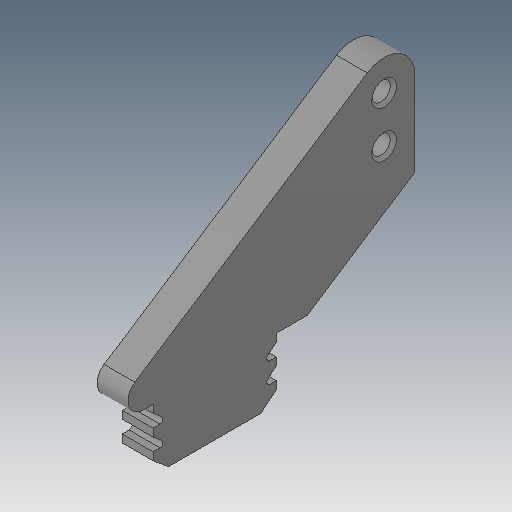
# Autodesk Inventor part: control_horn
Saved by Autodesk Inventor 2019 (Build 230136000, 136)
## iProperties
Created: 2022-04-02
Part Number: control_horn
Material: ABS Plastic
Document SubType Name: Modeling
Designer: solyo
Density: 1.06 g/cm^3
Appearance: Smooth - Medium Gray
Mass: 0.317862 g
Surface Area: 4.33026 cm^2
Volume: 0.29987 cm^3
Author: solyo
Autodesk Inventor part; units mm, degrees
ref_plane "YZ Plane" through (0, 0, 0) normal (1, 0, 0) x (0, 1, 0)
ref_plane "XZ Plane" through (0, 0, 0) normal (0, 1, 0) x (-1, 0, 0)
ref_plane "XY Plane" through (0, 0, 0) normal (0, 0, 1) x (1, 0, 0)
sketch "Sketch1" plane through (0, 0, 0) normal (1, 0, 0) x (0, 1, 0)
  line L0 (0, 0) -> (11.6754, -17.9077)
  line L1 (10, -21) -> (4.5638, -21)
  line L2 (0, -14) -> (4.5638, -21)
  line L3 (0, 0) -> (0, -4)
  line L4 (0, -4) -> (-4, -4)
  line L5 (-4, -4) -> (-4, -12)
  line L6 (-4, -12) -> (0, -12)
  line L7 (0, -12) -> (0, -14)
  arc A0 (10, -21) -> (11.6754, -17.9077) centre (10, -19) ccw
  point P0 (13.6915, -21)
  point P1 (7, -19)
  dimension "d26" = 8
  dimension "d31" = 4
  dimension "d32" = 2
  dimension "d43" = 2
  dimension "d44" = 5
  dimension "d45" = 10
  dimension "d64" = 3
  dimension "d65" = 4
  constraints: 16 end point, 3 parallel, 3 point on line, 2 horizontal, 2 point on circle, 2 tangent, 1 centre point, 1 coincident, 1 collinear, 1 vertical
  measures "d26" distance of L4.end L5.end
  measures "d31" distance between parallel lines of L3 L5
  measures "d32" distance of L6.end L2.start
  measures "d43" radius of A0
  measures "d44" vertical distance of L2.start A0.centre
  measures "d45" horizontal distance of L0.start point (10, -19)
  measures "d64" distance of A0.centre point (7, -19)
  measures "d65" distance of L0.start L3.end
extrude "Extrusion1" add sketch "Sketch1" along normal blind 2
hole "Hole3" at (0, 10, -19) at (0, 7, -19) direction (1, 0, 0) diameter 1.2 end through all
fillet "Fillet3" radius 1 1 edges at (1, 0, 0)
chamfer "Chamfer2" distance 0.2 angle 45 4 edges at (2, 10, -19.6) (0, 10, -19.6) (0, 7, -19.6) (2, 7, -19.6)
ref_plane "Work Plane1" through (0, -4, -8) normal (0, 0, -1) x (-1, 0, 0)
sketch "Sketch4" plane through (2, 0, 0) normal (1, 0, 0) x (0, 0, -1)
  arc A0 (2.8186, 1.8377) -> (3.3648, 0) centre (3.3648, 1) ccw projected
  line L0 (3.3648, 0) -> (4, 0) projected
  line L1 (4, 0) -> (4, -4) projected
  line L2 (4, -4) -> (12, -4) projected
  line L3 (12, -4) -> (12, 0) projected
  line L4 (12, 0) -> (14, 0) projected
  line L5 (14, 0) -> (21, 4.5638) projected
  line L6 (21, 4.5638) -> (21, 10) projected
  arc A1 (21, 10) -> (17.9077, 11.6754) centre (19, 10) ccw projected
  line L7 (17.9077, 11.6754) -> (2.8186, 1.8377) projected
  circle A2 centre (19, 10) radius 0.8 projected
  line L8 (4, 0) -> (12, 0)
  line L9 (12, -4) -> (4, -4) projected
  line L10 (5, -4) -> (4, -3.1667)
  line L11 (4, -4) -> (4, 0) projected
  line L12 (4, -2.6667) -> (5, -2.6667)
  line L13 (5, -2.6667) -> (4, -1.8333)
  line L14 (4, -1.3333) -> (5, -1.3333)
  line L15 (5, -1.3333) -> (4, -0.5)
  line L16 (4, -0.5) -> (4, 0)
  line L17 (4, -0.5) -> (4, -1.3333)
  line L18 (4, -1.8333) -> (4, -2.6667)
  line L19 (4, -3.1667) -> (4, -4)
  line L20 (4, -4) -> (5, -4)
  point P0 (0, 0)
  dimension "d57" = 1
  dimension "d58" = 0.5
  dimension "d59" = 0.5
  dimension "d60" = 0.5
  constraints: 22 end point, 6 point on line, 3 collinear, 3 perpendicular, 2 parallel, 2 vertical alignment, 1 horizontal, 1 vertical
  measures "d57" distance of L1.end L10.start
  measures "d58" distance of L13.end L14.start
  measures "d59" distance of L12.start L10.end
  measures "d60" distance of L15.end L0.end
extrude "Extrusion2" cut sketch "Sketch4" against normal through all contours L15 L14 L1 | L13 L12 L1 | L2 L1 L10
mirror "Mirror1" about plane through (0, -4, -8) normal (0, 0, -1) of "Extrusion2"
fillet "Fillet4" radius 0.2 4 edges at (1, -1.3333, -11) (1, -2.6667, -11) (1, -1.3333, -5) (1, -2.6667, -5)
equation "\"d59\" = d58"
equation "\"d60\" = d58"
equation "\"d1\" = d0"
equation "\"d21\" = d1"
equation "\"d0\" = 12"
body "Solid1"
